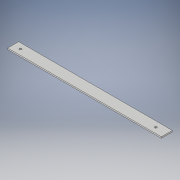
# Autodesk Inventor part: Hard Stop
Saved by Autodesk Inventor 2018.3 (Build 223284000, 284)
## iProperties
Created: 2019-03-03
Part Number: Hard Stop
Material: Generic
Document SubType Name: Modeling
Designer: Refraction
Density: 1 g/cm^3
Appearance: Default
Author: Refraction
Autodesk Inventor part; units mm, degrees
ref_plane "YZ Plane" through (0, 0, 0) normal (1, 0, 0) x (0, 1, 0)
ref_plane "XZ Plane" through (0, 0, 0) normal (0, 1, 0) x (-1, 0, 0)
ref_plane "XY Plane" through (0, 0, 0) normal (0, 0, 1) x (1, 0, 0)
sketch "Sketch1" plane through (0, 0, 0) normal (0, 1, 0) x (-1, 0, 0)
  line L0 (0, 0) -> (355.6, 0)
  line L1 (355.6, 0) -> (355.6, -25.4)
  line L2 (355.6, -25.4) -> (0, -25.4)
  line L3 (0, -25.4) -> (0, 0)
  dimension "d0" = 355.6
  dimension "d1" = 25.4
  constraints: 8 end point, 2 parallel, 1 horizontal, 1 perpendicular
  measures "d0" distance of L1.end L2.end
  measures "d1" distance of L0.end L1.end
extrude "Extrusion1" add sketch "Sketch1" along normal blind 3.175
sketch "Sketch2" plane through (0, 3.175, 0) normal (0, 1, 0) x (1, 0, 0)
  line L0 (0, 0) -> (0, 25.4) construction
  line L1 (0, 12.7) -> (-25.4, 12.7) construction
  line L2 (-25.4, 12.7) -> (-338.709, 12.7) construction
  circle A0 centre (-25.4, 12.7) radius 2.5797
  circle A1 centre (-338.709, 12.7) radius 2.5797
  dimension "d4" = 25.4
  dimension "d5" = 313.309
  dimension "d6" = 5.1594
  dimension "d7" = 5.1594
  constraints: 4 end point, 2 centre point, 2 coincident, 2 horizontal, 1 midpoint
  measures "d4" distance of L1.start L1.end
  measures "d5" distance of L1.end L2.end
  measures "d6" diameter of A0
  measures "d7" diameter of A1
extrude "Extrusion2" cut sketch "Sketch2" against normal blind 3.175
body "Solid1"
